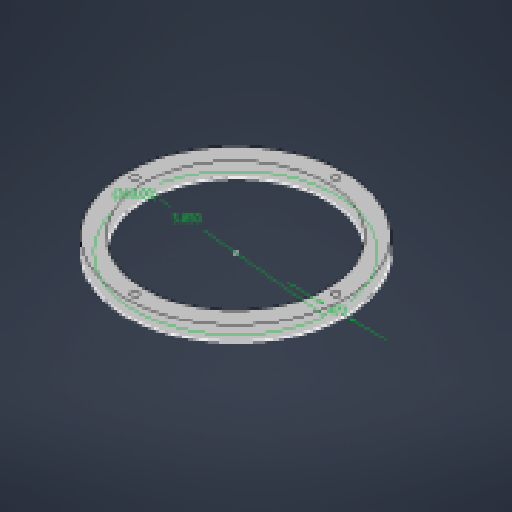
# Autodesk Inventor part: OR
Saved by Autodesk Inventor 2024 (Build 280153000, 153)
## iProperties
Created: 2023-10-21
Part Number: OR
Material: Generic
Document SubType Name: Modeling
Designer: range
Density: 1 g/cm^3
Appearance: Default
Author: range
Autodesk Inventor part; units mm, degrees
ref_plane "YZ Plane" through (0, 0, 0) normal (1, 0, 0) x (0, 1, 0)
ref_plane "XZ Plane" through (0, 0, 0) normal (0, 1, 0) x (-1, 0, 0)
ref_plane "XY Plane" through (0, 0, 0) normal (0, 0, 1) x (1, 0, 0)
sketch "Sketch1" plane through (0, 0, 0) normal (0, 1, 0) x (-1, 0, 0)
  circle A0 centre (0, 0) radius 74.3
  circle A1 centre (0, 0) radius 62.3
  line L0 (62.3, 0) -> (74.3, 0) construction
  point P0 (68.3, 0)
  point P1 (0, 68.3)
  point P2 (-68.3, 0)
  point P3 (0, -68.3)
  dimension "d0" = 148.6
  dimension "d1" = 12
  dimension "d4" = 360
  constraints: 2 end point, 2 horizontal alignment, 1 coincident, 1 horizontal, 1 midpoint, 1 point on line, 9 other
extrude "Extrusion1" add sketch "Sketch1" along normal blind 10
hole "Hole1" at (-68.3, 0, 0) at (0, 0, 68.3) at (68.3, 0, 0) at (0, 0, -68.3) direction (0, 1, 0) diameter 5 end through all countersink diameter 10.3886 countersink angle 90 clearance for "Flat Head Machine Screw" size "M5" standard "Ansi Metric M Profile"
body "Solid1"
